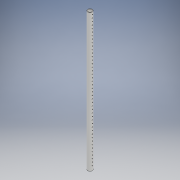
# Autodesk Inventor part: Ground_Antenna230mm_Support
Saved by Autodesk Inventor 2018 (Build 220112000, 112)
## iProperties
Created: 2018-10-12
Part Number: Ground_Antenna230mm_Support
Material: PVC-Piping
Document SubType Name: Modeling
Designer: Bradley
Density: 1.4 g/cm^3
Appearance: Smooth - White
Mass: 617.957 g
Surface Area: 2284.9 cm^2
Volume: 441.398 cm^3
Author: Bradley
Autodesk Inventor part; units mm, degrees
ref_plane "YZ Plane" through (0, 0, 0) normal (1, 0, 0) x (0, 1, 0)
ref_plane "XZ Plane" through (0, 0, 0) normal (0, 1, 0) x (-1, 0, 0)
ref_plane "XY Plane" through (0, 0, 0) normal (0, 0, 1) x (1, 0, 0)
sketch "Sketch1" plane through (0, 0, 0) normal (0, 0, 1) x (1, 0, 0)
  circle A0 centre (0, 0) radius 21.082
  circle A1 centre (0, 0) radius 17.526
  dimension "d0" = 42.164
  dimension "d1" = 35.052
  constraints: 2 centre point, 2 coincident
  measures "d0" diameter of A0
  measures "d1" diameter of A1
extrude "Extrusion1" add sketch "Sketch1" along normal mid plane 1225
sketch "Sketch2" plane through (0, 0, 0) normal (1, 0, 0) x (0, 1, 0)
  line L0 (17.526, -612.5) -> (-17.526, -612.5) projected
  line L1 (17.526, -612.5) -> (-17.526, -612.5) projected
  line L2 (-17.526, 612.5) -> (17.526, 612.5) projected
  line L3 (-21.082, -612.5) -> (-21.082, 612.5) projected
  point P0 (0, 0)
  point P1 (0, -573.9792)
  point P2 (0, -612.5)
  point P3 (0, -546.8293)
  point P4 (0, -519.6792)
  point P5 (0, -492.5292)
  point P6 (0, -465.3792)
  point P7 (0, -438.2292)
  point P8 (0, -411.0792)
  point P9 (0, -383.9292)
  point P10 (0, -356.7792)
  point P11 (0, -329.6292)
  point P12 (0, -302.4792)
  point P13 (0, -275.3292)
  point P14 (0, -248.1792)
  point P15 (0, -221.0292)
  point P16 (0, -193.8792)
  point P17 (0, -166.7292)
  point P18 (0, -139.5792)
  point P19 (0, -112.4292)
  point P20 (0, -85.2792)
  point P21 (0, -58.1292)
  point P22 (0, -30.9792)
  point P23 (0, -3.8292)
  point P24 (0, 23.3208)
  point P25 (0, 50.4708)
  point P26 (0, 77.6208)
  point P27 (0, 104.7708)
  point P28 (0, 131.9208)
  point P29 (0, 159.0708)
  point P30 (0, 186.2208)
  point P31 (0, 213.3708)
  point P32 (0, 240.5208)
  point P33 (0, 267.6708)
  point P34 (0, 294.8208)
  point P35 (0, 321.9708)
  point P36 (0, 349.1208)
  point P37 (0, 376.2708)
  point P38 (0, 403.4208)
  point P39 (0, 430.5708)
  point P40 (0, 457.7208)
  point P41 (0, 484.8708)
  point P42 (0, 512.0208)
  point P43 (0, 539.1708)
  point P44 (0, 566.3208)
  point P45 (0, 593.4708)
  dimension "d4" = 38.5207
  dimension "d7" = 27.15
  constraints: 1 midpoint, 1 vertical, 1 vertical alignment, 43 other
  measures "d4" distance from line of L0 point (0, -573.979)
  measures "d7" distance of point (0, -573.979) point (0, -546.829)
hole "Hole1" at (0, 0, -573.9792) at (0, 0, -546.8293) at (0, 0, -519.6792) at (0, 0, -492.5292) at (0, 0, -465.3792) at (0, 0, -438.2292) at (0, 0, -411.0792) at (0, 0, -383.9292) at (0, 0, -356.7792) at (0, 0, -329.6292) at (0, 0, -302.4792) at (0, 0, -275.3292) at (0, 0, -248.1792) at (0, 0, -221.0292) at (0, 0, -193.8792) at (0, 0, -166.7292) at (0, 0, -139.5792) at (0, 0, -112.4292) at (0, 0, -85.2792) at (0, 0, -58.1292) at (0, 0, -30.9792) at (0, 0, -3.8292) at (0, 0, 23.3208) at (0, 0, 50.4708) at (0, 0, 77.6208) at (0, 0, 104.7708) at (0, 0, 131.9208) at (0, 0, 159.0708) at (0, 0, 186.2208) at (0, 0, 213.3708) at (0, 0, 240.5208) at (0, 0, 267.6708) at (0, 0, 294.8208) at (0, 0, 321.9708) at (0, 0, 349.1208) at (0, 0, 376.2708) at (0, 0, 403.4208) at (0, 0, 430.5708) at (0, 0, 457.7208) at (0, 0, 484.8708) at (0, 0, 512.0208) at (0, 0, 539.1708) at (0, 0, 566.3208) at (0, 0, 593.4708) direction (-1, 0, 0) diameter 6.35 end through all both
body "Solid1"
